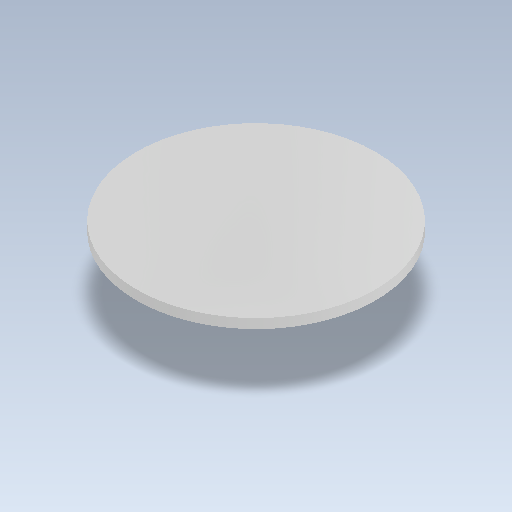
# Autodesk Inventor part: mirror_50
Saved by Autodesk Inventor 2020 (Build 240168000, 168)
## iProperties
Created: 2024-02-27
Part Number: mirror_50
Material: Алюминий 6061-AHC
Document SubType Name: Modeling
Designer: 4s
Density: 2.7 g/cm^3
Appearance: Алюминий — полированный
Author: 4s
Autodesk Inventor part; units mm, degrees
ref_plane "YZ Plane" through (0, 0, 0) normal (1, 0, 0) x (0, 1, 0)
ref_plane "XZ Plane" through (0, 0, 0) normal (0, 1, 0) x (-1, 0, 0)
ref_plane "XY Plane" through (0, 0, 0) normal (0, 0, 1) x (1, 0, 0)
sketch "Эскиз1" plane through (0, 0, 0) normal (1, 0, 0) x (0, 1, 0)
  line L0 (0, 0) -> (0, -25)
  line L1 (0, 0) -> (-61.7134, 0) construction
  line L2 (0, 0) -> (0, 25)
  line L3 (-2, 25) -> (-2, -25)
  line L4 (0, 25) -> (-2, 25)
  line L5 (0, -25) -> (-2, -25)
  line L6 (-3.5, 17.5) -> (-3.5, -17.5)
  line L7 (-3.5, 17.5) -> (-2, 17.5)
  line L8 (-3.5, -17.5) -> (-2, -17.5)
  line L9 (-3.5, 17.5) -> (-12.1603, 2.5)
  line L10 (-3.5, -17.5) -> (-12.1603, -2.5)
  arc A0 (-12.1603, 2.5) -> (-12.1603, -2.5) centre (-7.8301, 0) ccw
  line L11 (0, 0) -> (-12.8301, 0)
  point P0 (-13.6036, 0)
  dimension "d0" = 50
  dimension "d1" = 2
  dimension "d2" = 35
  dimension "d3" = 1.5
  dimension "d4" = 30
  dimension "d5" = 5
  constraints: 24 end point, 7 point on line, 3 horizontal, 3 point on circle, 3 symmetric about line, 2 parallel, 2 tangent, 1 centre point, 1 perpendicular, 1 vertical
  measures "d0" distance of L0.end L2.end
  measures "d1" distance of L2.end L4.end
  measures "d2" distance of L6.start L6.end
  measures "d3" distance of L6.start L7.end
  measures "d4" angle of L6 L9
  measures "d5" radius of A0
revolve "Вращение1" add sketch "Эскиз1" angle 360 about axis through (0, 0, 0) along (0, -1, 0) contours L0 L5 L3 L11 | L3 L8 L6 L11 | L6 L10 A0 L11
